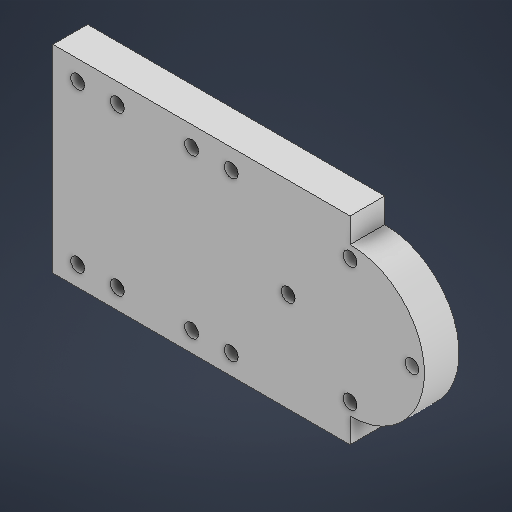
# Autodesk Inventor part: üst döner tablo1
Saved by Autodesk Inventor 2026.1 (Build 301233020, 233B)
## iProperties
Created: 2026-04-16
Part Number: üst döner tablo1
Material: Generic
Document SubType Name: Modeling
Designer: kadir
Density: 1 g/cm^3
Appearance: Default
Author: kadir
Autodesk Inventor part; units mm, degrees
ref_plane "YZ Plane" through (0, 0, 0) normal (1, 0, 0) x (0, 1, 0)
ref_plane "XZ Plane" through (0, 0, 0) normal (0, 1, 0) x (-1, 0, 0)
ref_plane "XY Plane" through (0, 0, 0) normal (0, 0, 1) x (1, 0, 0)
sketch "Sketch1" plane through (0, 0, 0) normal (0, 0, 1) x (1, 0, 0)
  line L0 (0, 0) -> (60, 0)
  line L1 (60, 0) -> (60, 40)
  line L2 (60, 40) -> (0, 40)
  line L3 (0, 40) -> (0, 0)
  circle A0 centre (60, 20) radius 15
  circle A1 centre (47.5, 20) radius 1.4
  circle A2 centre (60, 7.5) radius 1.4
  circle A3 centre (72.5, 20) radius 1.4
  circle A4 centre (60, 32.5) radius 1.4
  point P0 (60, 5)
  point P1 (60, 35)
  dimension "d0" = 60
  dimension "d1" = 40
  dimension "d2" = 30
  dimension "d3" = 2.8
  dimension "d4" = 12.5
  dimension "d7" = 360
  constraints: 8 end point, 5 centre point, 2 parallel, 1 coincident, 1 horizontal, 1 midpoint, 1 perpendicular, 9 other
  measures "d0" distance of L2.end L1.end
  measures "d1" distance of L1.end L0.end
  measures "d2" diameter of A0
  measures "d3" diameter of A1
  measures "d4" distance of A1.centre A0.centre
extrude "Extrusion1" add sketch "Sketch1" along normal blind 7 contours L3 L2 L1 A0 L0 | A0 L1 A4 A2 | L1 A2 A4 A0
sketch "Sketch2" plane through (0, 0, 7) normal (0, 0, 1) x (1, 0, 0)
  line L0 (13, 36) -> (36, 36)
  line L1 (36, 36) -> (36, 4)
  line L2 (36, 4) -> (13, 4)
  line L3 (13, 4) -> (13, 36)
  line L4 (0, 40) -> (0, 0) projected
  circle A0 centre (13, 36) radius 1.4
  line L5 (0, 20) -> (36, 20)
  circle A1 centre (13, 4) radius 1.4
  line L6 (24.5, 36) -> (24.5, 4)
  circle A2 centre (36, 36) radius 1.4
  circle A3 centre (36, 4) radius 1.4
  dimension "d11" = 23
  dimension "d12" = 32
  dimension "d13" = 2.8
  dimension "d22" = 13
  constraints: 12 end point, 4 centre point, 4 midpoint, 3 symmetric about line, 2 parallel, 2 perpendicular, 1 coincident, 1 horizontal, 1 horizontal alignment, 3 other
  measures "d11" distance of L1.end L2.end
  measures "d12" distance of L0.end L1.end
  measures "d13" diameter of A0
  measures "d22" distance from line of L4 A0.centre
extrude "Extrusion2" cut sketch "Sketch2" against normal through all contours L3 A0 L0 | L0 A0 L3 | A2 L1 L0 | L0 L1 A2 | A1 L2 L3 | L3 L2 A1 | A3 L2 L1 | L1 L2 A3
sketch "Sketch3" plane through (0, 0, 7) normal (0, 0, 1) x (1, 0, 0)
  line L0 (5, 36) -> (28, 36)
  line L1 (28, 36) -> (28, 4)
  line L2 (28, 4) -> (5, 4)
  line L3 (5, 4) -> (5, 36)
  line L4 (0, 40) -> (0, 0) projected
  circle A0 centre (36, 36) radius 1.4 projected
  circle A1 centre (5, 36) radius 1.4
  line L5 (0, 20) -> (28, 20)
  circle A2 centre (5, 4) radius 1.4
  line L6 (16.5, 36) -> (16.5, 4)
  circle A3 centre (28, 36) radius 1.4
  circle A4 centre (28, 4) radius 1.4
  point P0 (5, 20)
  dimension "d16" = 23
  dimension "d17" = 32
  dimension "d18" = 8
  dimension "d19" = 2.8
  constraints: 12 end point, 5 midpoint, 4 centre point, 3 symmetric about line, 2 parallel, 1 coincident, 1 horizontal, 1 horizontal alignment, 1 perpendicular, 3 other
  measures "d16" distance of L1.end L2.end
  measures "d17" distance of L0.end L1.end
  measures "d18" distance of A0.centre L0.end
  measures "d19" diameter of A1
extrude "Extrusion3" cut sketch "Sketch3" against normal through all contours L3 A1 L0 | L0 A1 L3 | A3 L1 L0 | L0 L1 A3 | A2 L2 L3 | L3 L2 A2 | A4 L2 L1 | L1 L2 A4
body "Solid1"
